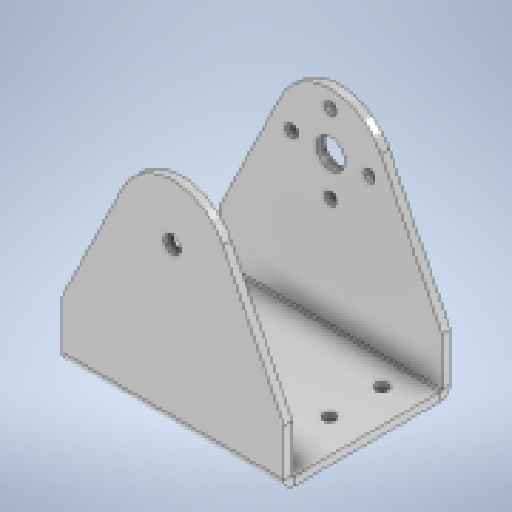
# Autodesk Inventor part: partpart
Saved by Autodesk Inventor 2025.2 (Build 292293000, 293)
## iProperties
Created: 2025-07-22
Part Number: partpart
Material: Aluminum 6061-AHC
Document SubType Name: Sheet Metal
Designer: User
Density: 2.7 g/cm^3
Sheet Metal Rule: Default_mm
Appearance: Aluminum - Dark
Author: User
Autodesk Inventor part; units mm, degrees
ref_plane "YZ Plane" through (0, 0, 0) normal (1, 0, 0) x (0, 1, 0)
ref_plane "XZ Plane" through (0, 0, 0) normal (0, 1, 0) x (-1, 0, 0)
ref_plane "XY Plane" through (0, 0, 0) normal (0, 0, 1) x (1, 0, 0)
sketch "Sketch1" plane through (0, 0, 0) normal (0, 1, 0) x (-1, 0, 0)
  line L0 (20, 14.965) -> (-20, 14.965)
  line L1 (-20, 14.965) -> (-20, -14.965)
  line L2 (-20, -14.965) -> (20, -14.965)
  line L3 (20, -14.965) -> (20, 14.965)
  point P0 (0, 0)
  dimension "d0" = 29.93
  dimension "d1" = 40
  dimension "d2" = 20
  dimension "d3" = 14.965
  measures "d0" distance of L2.end L0.start
  measures "d1" distance of L0.start L0.end
  measures "d2" distance from line of point (0, 0) L3
  measures "d3" distance from line of point (0, 0) L2
extrude "Plate1" add sketch "Sketch1" along normal blind 1.5
sketch "Sketch2" plane through (-20, 0, -13.465) normal (0, 0, -1) x (-1, 0, 0)
  line L0 (-40, 0) -> (0, 0)
  line L1 (0, 0) -> (0, 38.5)
  line L2 (0, 38.5) -> (-40, 38.5)
  line L3 (-40, 38.5) -> (-40, 0)
  constraints: 6 end point, 1 horizontal, 1 perpendicular, 1 vertical
edge flange "Flange1" height 38.5 angle 90 thickness 1.5 bend radius 0.31 thickness toward (0, 0, -1) relief tear relief width 1.5 relief depth 0.75 corner gap 0.31 corner form 0 edges at (0, 1.5, -14.965) (0, 1.5, 14.965) wall of the first edge with corners at (20, 0, -13.465) (-20, 0, -13.465) (-20, 38.5, -13.465) (20, 38.5, -13.465)
bend "Bend1"
corner "Corner1"
sketch "Sketch3" plane through (-20, 38.5, 14.965) normal (0, 0, 1) x (1, 0, 0)
  line L0 (0, 0) -> (40, 0) projected
  line L1 (0, -36.69) -> (0, 0) projected
  circle A0 centre (20, -10) radius 10
  line L2 (0, -28.19) -> (40, -28.19)
  line L3 (40, -28.19) -> (40, -38.19)
  line L4 (40, -38.19) -> (0, -38.19)
  line L5 (0, -38.19) -> (0, -28.19)
  line L6 (40, -28.19) -> (28.9876, -5.6156)
  line L7 (0, -28.19) -> (11.0124, -5.6156)
  line L8 (0, 0) -> (40, 0)
  line L9 (40, 0) -> (40, -35)
  line L10 (40, -35) -> (0, -35)
  line L11 (0, -35) -> (0, 0)
  point P0 (20, -38.5)
  point P1 (20, 0)
  point P2 (0, -28.19)
  point P3 (0, -35)
  point P4 (30, -10)
  dimension "d15" = 10
  dimension "d16" = 0
  dimension "d17" = 20
  dimension "d18" = 18.19
  dimension "d19" = 0
  dimension "d20" = 40
  dimension "d21" = 10
  dimension "d22" = 35
  constraints: 20 end point, 4 parallel, 2 horizontal, 2 perpendicular, 2 point on circle, 2 tangent, 1 centre point, 1 point on line
  measures "d15" distance from line of L0 A0.centre
  measures "d16" horizontal distance of point (20, -38.5) A0.centre
  measures "d17" diameter of A0
  measures "d18" distance from line of A0.centre L2
  measures "d19" distance between parallel lines of L1 L5
  measures "d20" distance of L3.end L4.end
  measures "d21" distance between parallel lines of L2 L4
  measures "d22" distance between parallel lines of L0 L10
extrude "Extrusion1" cut sketch "Sketch3" against normal blind 35 contours L0 A0 L7 L1 | L0 L9 L6 A0
sketch "Sketch4" plane through (20, 1.81, -14.965) normal (0, 0, -1) x (-1, 0, 0)
  arc A0 (28.9876, 31.0744) -> (11.0124, 31.0744) centre (20, 26.69) ccw projected
  circle A1 centre (20, 26.69) radius 2.6
  circle A2 centre (13, 26.69) radius 1.05
  circle A3 centre (27, 26.69) radius 1.05
  circle A4 centre (20, 33.69) radius 1.05
  circle A5 centre (20, 19.69) radius 1.05
  point P0 (20, -1.81)
  dimension "d25" = 5.2
  dimension "d26" = 0
  dimension "d27" = 7
  dimension "d28" = 2.1
  dimension "d29" = 7
  dimension "d30" = 0
  dimension "d31" = 2.1
  dimension "d32" = 0
  dimension "d33" = 7
  dimension "d34" = 2.1
  dimension "d35" = 7
  dimension "d36" = 0
  dimension "d37" = 2.1
  constraints: 5 centre point, 1 coincident
  measures "d25" diameter of A1
  measures "d26" vertical distance of A0.centre A2.centre
  measures "d27" distance of A0.centre A2.centre
  measures "d28" diameter of A2
  measures "d29" distance of A4.centre A0.centre
  measures "d30" horizontal distance of A0.centre A4.centre
  measures "d31" diameter of A4
  measures "d32" vertical distance of A0.centre A3.centre
  measures "d33" distance of A0.centre A3.centre
  measures "d34" diameter of A3
  measures "d35" distance of A0.centre A5.centre
  measures "d36" horizontal distance of A0.centre A5.centre
  measures "d37" diameter of A5
extrude "Extrusion2" cut sketch "Sketch4" against normal blind 1.5
sketch "Sketch5" plane through (-20, 1.81, 14.965) normal (0, 0, 1) x (1, 0, 0)
  arc A0 (28.9876, 31.0744) -> (11.0124, 31.0744) centre (20, 26.69) ccw projected
  circle A1 centre (20, 26.69) radius 1.5
  point P0 (20, -1.81)
  dimension "d40" = 3
  constraints: 1 centre point, 1 coincident
  measures "d40" diameter of A1
extrude "Extrusion3" cut sketch "Sketch5" against normal blind 1.5
sketch "Sketch6" plane through (0, 1.5, 0) normal (0, 1, 0) x (1, 0, 0)
  circle A0 centre (-14, -10.155) radius 1.05 projected
  circle A1 centre (-14, -0.75) radius 1.05 projected
  circle A2 centre (-14, 8.655) radius 1.05 projected
  circle A3 centre (14, -10.155) radius 1.05 projected
  circle A4 centre (14, -0.75) radius 1.05 projected
  circle A5 centre (14, 8.655) radius 1.05 projected
  point P0 (0, 0)
hole "Hole1" at (14, 1.5, -8.655) at (14, 1.5, 0.75) at (14, 1.5, 10.155) at (-14, 1.5, 10.155) at (-14, 1.5, 0.75) at (-14, 1.5, -8.655) direction (0, -1, 0) diameter 2.1 depth 1.5
equation "\"d48\" = Thickness"
equation "\"d4\" = Thickness"
equation "\"d5\" = BendReliefWidth"
equation "\"d6\" = BendReliefDepth"
equation "\"d7\" = MinimumRemnant"
equation "\"d8\" = TransitionRadius"
equation "\"d11\" = BendRadius"
equation "\"d12\" = CornerReliefSize"
equation "\"d13\" = GapSize"
equation "\"d14\" = JacobiRadiusSize"
equation "\"BendReliefWidth\" = Thickness"
equation "\"BendReliefDepth\" = 0.5 * Thickness"
equation "\"CornerReliefSize\" = 4 * Thickness"
equation "\"MinimumRemnant\" = 2 * Thickness"
equation "\"TransitionRadius\" = BendRadius"
equation "\"JacobiRadiusSize\" = BendRadius"
equation "\"GapSize\" = Thickness"
equation "\"Thickness\" = 1.5"
equation "\"BendRadius\" = 0.31"
body "Solid1"
